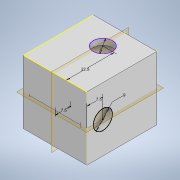
# Autodesk Inventor part: extruder mount
Saved by Autodesk Inventor 2020 (Build 240168000, 168)
## iProperties
Created: 2021-03-16
Part Number: extruder mount
Material: Generic
Document SubType Name: Modeling
Designer: AOB
Mass: 20.3864 g
Surface Area: 85.7047 cm^2
Volume: 20.3864 cm^3
Density: 1 g/cm^3
Appearance: Default
Author: AOB
Autodesk Inventor part; units mm, degrees
ref_plane "YZ Plane" through (0, 0, 0) normal (1, 0, 0) x (0, 1, 0)
ref_plane "XZ Plane" through (0, 0, 0) normal (0, 1, 0) x (-1, 0, 0)
ref_plane "XY Plane" through (0, 0, 0) normal (0, 0, 1) x (1, 0, 0)
sketch "Sketch1" plane through (0, 0, 0) normal (0, 0, 1) x (1, 0, 0)
  line L0 (0, 0) -> (30, 0)
  line L1 (30, 0) -> (30, -30)
  line L2 (30, -30) -> (0, -30)
  line L3 (0, -30) -> (0, 0)
  dimension "d0" = 30
  dimension "d1" = 30
  constraints: 8 end point, 2 parallel, 1 horizontal, 1 perpendicular
  measures "d0" distance of L0.end L1.end
  measures "d1" distance of L1.end L2.end
extrude "Extrusion2" add sketch "Sketch1" along normal blind 33
ref_plane "Work Plane1" through (0, 0, 16.5) normal (0, 0, -1) x (-1, 0, 0)
sketch "Sketch3" plane through (0, 0, 0) normal (0, 1, 0) x (1, 0, 0)
  line L0 (0, 0) -> (0, -33) projected
  circle A0 centre (15, -10.5) radius 4.5
  line L1 (30, -33) -> (0, -33) projected
  dimension "d11" = 9
  dimension "d23" = 22.5
  constraints: 1 centre point
  measures "d11" diameter of A0
  measures "d23" distance from line of L1 A0.centre
ref_plane "Work Plane3" through (0, -15, 0) normal (0, 1, 0) x (1, 0, 0)
sketch "Sketch4" plane through (0, -15, 0) normal (0, 1, 0) x (1, 0, 0)
  circle A0 centre (15, -10.5) radius 7.5
  line L0 (0, -33) -> (30, -33) projected
  line L1 (0, 0) -> (0, -33) projected
  dimension "d24" = 22.5
  dimension "d25" = 15
  constraints: 1 centre point, 1 coincident
  measures "d24" distance from line of L0 point (15, -10.5)
  measures "d25" distance from line of L1 point (15, -10.5)
extrude "Extrusion4" cut sketch "Sketch4" along normal mid plane 24.3
extrude "Extrusion5" cut sketch "Sketch3" against normal through all
sketch "Sketch5" plane through (30, -30, 0) normal (1, 0, 0) x (0, 0, -1)
  line L0 (-33, 0) -> (-33, 30) construction
  line L1 (-33, 15) -> (-25.5, 15) construction
  circle A0 centre (-25.5, 15) radius 4.5
  point P0 (0, 30)
  dimension "d16" = 7.5
  dimension "d17" = 9
  constraints: 2 end point, 1 centre point, 1 coincident, 1 horizontal, 1 midpoint
  measures "d16" distance of L1.start L1.end
  measures "d17" diameter of A0
extrude "Extrusion6" cut sketch "Sketch5" against normal through all
ref_plane "Work Plane4" through (15, -30, 0) normal (1, 0, 0) x (0, 0, -1)
sketch "Sketch6" plane through (15, -30, 0) normal (1, 0, 0) x (0, 0, -1)
  line L0 (-33, 15) -> (-25.5, 15) construction
  circle A0 centre (-25.5, 15) radius 7.5
  point P0 (0, 30)
  dimension "d20" = 7.5
  constraints: 2 end point, 1 coincident, 1 horizontal, 1 horizontal alignment, 2 other
  measures "d20" distance of L0.start L0.end
extrude "Extrusion7" cut sketch "Sketch6" along normal mid plane 24.3
body "Solid2"
